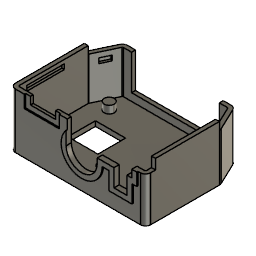
logger_case_bottom (Autodesk Fusion 360 design; units mm, degrees)
part number: 2026-07-28-14-06-36-773
Autodesk Fusion 360 part; units mm, degrees
sketch "Skizze1" plane through (0, 0, 0) normal (0, 0, 1) x (1, 0, 0)
  line L0 (0, 0) -> (-54, 0)
  line L1 (-54, 0) -> (-54, 30)
  line L2 (-54, 30) -> (-49, 40.5)
  line L3 (-49, 40.5) -> (-5, 40.5)
  line L4 (-5, 40.5) -> (0, 30)
  line L5 (0, 30) -> (0, 0)
  dimension "d1" = 54
  dimension "d2" = 30
  dimension "d3" = 40.5
  dimension "d4" = 30
  dimension "d5" = 10.5
  dimension "d6" = 44
  dimension "d7" = 5
  dimension "d8" = 5
  constraint coincident L0.start L5.end
  constraint horizontal L0
  constraint perpendicular L0 L1
  constraint perpendicular L1 L3
  constraint perpendicular L0 L5
  measures "d1" distance of L0.start L0.end
  measures "d2" distance of L0.end L1.end
  measures "d3" distance of L0 L3
  measures "d4" distance of L0.start L4.end
  measures "d5" distance of L3 L4.end
  measures "d6" distance of L2.end L3.end
  measures "d7" distance of L1 L2.end
  measures "d8" distance of L3.end L5
extrude "Extrusion1" add sketch "Skizze1" along normal blind 2 makes body 1
fillet "Abrundung1" radius 2 1 edges at (-54, 0, 1) on bodies 1
fillet "Abrundung2" radius 2 1 edges at (0, 0, 1) on bodies 1
fillet "Abrundung3" radius 2 1 edges at (0, 30, 1) on bodies 1
fillet "Abrundung4" radius 2 1 edges at (-5, 40.5, 1) on bodies 1
fillet "Abrundung5" radius 2 1 edges at (-49, 40.5, 1) on bodies 1
fillet "Abrundung6" radius 2 1 edges at (-54, 30, 1) on bodies 1
sketch "Skizze2" plane through (0, 0, 2) normal (0, 0, 1) x (-1, 0, 0)
  arc A0 (53.8057, -30.408) -> (54, -29.5481) centre (52, -29.5481) ccw
  line L0 (54, -29.5481) -> (54, -2)
  arc A1 (54, -2) -> (52, 0) centre (52, -2) ccw
  line L1 (52, 0) -> (2, 0)
  arc A2 (2, 0) -> (0, -2) centre (2, -2) ccw
  line L2 (0, -2) -> (0, -29.5481)
  arc A3 (0, -29.5481) -> (0.1943, -30.408) centre (2, -29.5481) ccw
  line L3 (0.1943, -30.408) -> (4.4571, -39.3599)
  arc A4 (4.4571, -39.3599) -> (6.2628, -40.5) centre (6.2628, -38.5) ccw
  line L4 (6.2628, -40.5) -> (47.7372, -40.5)
  arc A5 (47.7372, -40.5) -> (49.5429, -39.3599) centre (47.7372, -38.5) ccw
  line L5 (49.5429, -39.3599) -> (53.8057, -30.408)
  line L6 (1.6389, -29.7201) -> (5.9017, -38.672)
  arc A6 (5.9017, -38.672) -> (6.2628, -38.9) centre (6.2628, -38.5) ccw
  line L7 (6.2628, -38.9) -> (47.7372, -38.9)
  arc A7 (47.7372, -38.9) -> (48.0983, -38.672) centre (47.7372, -38.5) ccw
  line L8 (48.0983, -38.672) -> (52.3611, -29.7201)
  arc A8 (52.3611, -29.7201) -> (52.4, -29.5481) centre (52, -29.5481) ccw
  line L9 (52.4, -29.5481) -> (52.4, -2)
  arc A9 (52.4, -2) -> (52, -1.6) centre (52, -2) ccw
  line L10 (52, -1.6) -> (2, -1.6)
  arc A10 (2, -1.6) -> (1.6, -2) centre (2, -2) ccw
  line L11 (1.6, -2) -> (1.6, -29.5481)
  arc A11 (1.6, -29.5481) -> (1.6389, -29.7201) centre (2, -29.5481) ccw
  dimension "d23" = -1.6
extrude "Extrusion2" add sketch "Skizze2" along normal blind 20 bodies 1
sketch "Skizze3" plane through (0, 0, 0) normal (0, -1, 0) x (1, 0, 0)
  line L0 (-52, 22) -> (-52, 0)
  line L1 (-52, 0) -> (-2, 0)
  line L2 (-52, 22) -> (-46.4, 22)
  line L3 (-46.4, 22) -> (-46.4, 19)
  line L4 (-46.4, 19) -> (-36.4, 19)
  line L5 (-36.4, 19) -> (-36.4, 22)
  line L6 (-36.4, 22) -> (-31.2, 22)
  line L7 (-31.2, 13) -> (-31.2, 22)
  circle A0 centre (-25, 13) radius 6.2
  line L8 (0, 18) -> (-5, 18)
  line L9 (-5, 18) -> (-5, 15)
  line L10 (-5, 15) -> (-6.9, 15)
  line L11 (-6.9, 15) -> (-6.9, 8)
  line L12 (-6.9, 8) -> (-12.1, 8)
  line L13 (-12.1, 8) -> (-12.1, 15)
  line L14 (-46.4, 22) -> (-36.4, 22)
  line L15 (-31.2, 22) -> (0, 22)
  line L16 (-18.8, 13) -> (-18.8, 15)
  line L17 (-18.8, 15) -> (-12.1, 15)
  line L18 (0, 22) -> (0, 18)
  line L19 (0, 0) -> (-54, 0)
  line L20 (-54, 22) -> (-54, 0)
  point P0 (-54, 22)
  dimension "d27" = 3
  dimension "d28" = 10
  dimension "d29" = 5.2
  dimension "d30" = 12.4
  dimension "d31" = 13
  dimension "d32" = 9
  dimension "d33" = 6.2
  dimension "d36" = 19
  dimension "d37" = 4
  dimension "d40" = 5
  dimension "d41" = 3
  dimension "d42" = 1.9
  dimension "d43" = 7
  dimension "d44" = 5.2
  dimension "d45" = 7
  dimension "d123" = 7.6
  dimension "d127" = 6.2
  dimension "d129" = 6.7
  dimension "d131" = 10
  dimension "d132" = 31.2
  dimension "d150" = 22
  dimension "d151" = 18.8
  dimension "d152" = 22.8
  dimension "d154" = 8
  constraint coincident L0.start L2.start
  constraint perpendicular L2 L3
  constraint perpendicular L3 L4
  constraint perpendicular L6 L7
  constraint perpendicular L8 L9
  constraint perpendicular L9 L10
  constraint perpendicular L10 L11
  constraint perpendicular L11 L12
  constraint perpendicular L12 L13
  constraint parallel L6 L14
  constraint coincident A0 L16.start
  constraint vertical L16
  constraint parallel L15 L19
  constraint parallel L6 L19
  constraint parallel L2 L19
  constraint parallel L15 L17
  constraint parallel L12 L19
  constraint parallel L9 L18
  measures "d27" distance of L2.end L3.end
  measures "d28" distance of L3.end L4.end
  measures "d29" distance of L5.end L6.end
  measures "d30" diameter of A0
  measures "d31" distance of L1 A0.centre
  measures "d32" distance of L6.end L7.start
  measures "d33" distance of L7.start A0.centre
  measures "d36" distance of L1 L4
  measures "d37" distance of L8.start L15.end
  measures "d40" distance of L8.start L8.end
  measures "d41" distance of L8.end L9.end
  measures "d42" distance of L9.end L10.end
  measures "d43" distance of L10.end L11.end
  measures "d44" distance of L11.end L12.end
  measures "d45" distance of L12.end L13.end
  measures "d123" distance of L3 P0
  measures "d127" distance of A0.centre L16
  measures "d129" horizontal distance of L13.end L16.end
  measures "d131" horizontal distance of L2.end L5.end
  measures "d132" distance of L6.end L15.end
  measures "d150" distance of L0.start L0.end
  measures "d151" distance of L16.start L18
  measures "d152" distance of L7.start L20
  measures "d154" distance of L12 L19
extrude "Extrusion3" cut sketch "Skizze3" against normal blind 4 contours L7 A0 L8 L9 L10 L11 L12 L13 L15 L16 L17 L18 bodies 1
extrude "Extrusion4" cut sketch "Skizze3" against normal blind 3 contours A0 bodies 1
extrude "Extrusion5" cut sketch "Skizze3" against normal blind 3 contours L3 L4 L5 L14 bodies 1
sketch "Skizze4" plane through (0, 40.5, 0) normal (0, 1, 0) x (-1, 0, 0)
  line L0 (47.7372, 0) -> (47.7372, 22)
  line L1 (47.7372, 22) -> (6.2628, 22)
  line L2 (6.2628, 22) -> (6.2628, 0)
  line L3 (6.2628, 0) -> (47.7372, 0)
  line L4 (9.4998, 5) -> (44.4998, 5)
  line L5 (44.4998, 5) -> (44.4998, 22)
  line L6 (9.4998, 22) -> (44.4998, 22)
  line L7 (9.4998, 5) -> (9.4998, 22)
  line L8 (49, 0) -> (5, 0)
  line L9 (54.0455, 0) -> (54.0455, 22) construction
  line L10 (0.0455, 22) -> (0.0455, 0) construction
  point P0 (4.4571, 22)
  dimension "d56" = 17
  dimension "d57" = 35
  dimension "d58" = 3.237
  dimension "d59" = 3.2374
  dimension "d122" = 5
  dimension "d148" = 9.4543
  dimension "d149" = 9.5457
  constraint coincident L1 L6.start
  constraint perpendicular L2 L4
  constraint coincident L1 L5.end
  constraint perpendicular L1 L5
  constraint perpendicular L6 L7
  measures "d56" distance of L4.end L5.end
  measures "d57" distance of L4.start L4.end
  measures "d58" distance of L1.end L6.start
  measures "d59" distance of L0.end L5.end
  measures "d122" distance of L4 L8
  measures "d148" distance of L7 L10
  measures "d149" distance of L5 L9
extrude "Extrusion6" cut sketch "Skizze4" against normal blind 3 contours L1 L4 L5 L6 L7 bodies 1
sketch "Skizze5" plane through (0, 0, 22) normal (0, 0, 1) x (-1, 0, 0)
  line L0 (9.4998, -40.5) -> (9.4998, -38.9)
  line L1 (9.4998, -38.9) -> (6.2628, -38.9)
  arc A0 (5.9017, -38.672) -> (6.2628, -38.9) centre (6.2628, -38.5) ccw
  arc A1 (1.6, -29.5481) -> (1.6389, -29.7201) centre (2, -29.5481) ccw
  line L2 (1.6, -29.5481) -> (1.6, -4)
  line L3 (0, -4) -> (0, -29.5481)
  arc A2 (0, -29.5481) -> (0.1943, -30.408) centre (2, -29.5481) ccw
  line L4 (0.1943, -30.408) -> (4.4571, -39.3599)
  arc A3 (4.4571, -39.3599) -> (6.2628, -40.5) centre (6.2628, -38.5) ccw
  line L5 (6.2628, -40.5) -> (9.4998, -40.5)
  arc A4 (0, -29.5481) -> (0.1943, -30.408) centre (2, -29.5481) ccw
  line L6 (0.1943, -30.408) -> (4.4571, -39.3599)
  line L7 (49.5429, -39.3599) -> (53.8057, -30.408)
  arc A5 (53.8057, -30.408) -> (54, -29.5481) centre (52, -29.5481) ccw
  line L8 (44.4998, -40.5) -> (9.4998, -40.5)
  line L9 (44.4998, -40.5) -> (47.7372, -40.5)
  arc A6 (47.7372, -40.5) -> (49.5429, -39.3599) centre (47.7372, -38.5) ccw
  line L10 (6.2628, -40.5) -> (9.4998, -40.5)
  arc A7 (4.4571, -39.3599) -> (6.2628, -40.5) centre (6.2628, -38.5) ccw
  line L11 (54, -29.5481) -> (0, -29.5481)
  arc A8 (0, -29.5481) -> (0.1943, -30.408) centre (2, -29.5481) ccw
  line L12 (4.4571, -39.3599) -> (0.1943, -30.408)
  line L13 (1.6, -4) -> (0, -4)
  point P0 (0, -29.5481)
  constraint coincident A5.end L11.start
  constraint coincident P0 L3.end
extrude "Extrusion7" cut sketch "Skizze5" against normal blind 3 contours A2 L4 A3 L5 A4 L6 L7 A5 L8 L9 A6 L10 A7 L11 A8 L12 bodies 1
sketch "Skizze6" plane through (0, 0, 2) normal (0, 0, 1) x (-1, 0, 0)
  line L0 (1.6389, -29.7201) -> (5.9017, -38.672)
  arc A0 (5.9017, -38.672) -> (6.2628, -38.9) centre (6.2628, -38.5) ccw
  line L1 (6.2628, -38.9) -> (47.7372, -38.9)
  arc A1 (47.7372, -38.9) -> (48.0983, -38.672) centre (47.7372, -38.5) ccw
  line L2 (48.0983, -38.672) -> (52.3611, -29.7201)
  arc A2 (52.3611, -29.7201) -> (52.4, -29.5481) centre (52, -29.5481) ccw
  line L3 (52.4, -29.5481) -> (52.4, -2)
  arc A3 (52.4, -2) -> (52, -1.6) centre (52, -2) ccw
  line L4 (52, -1.6) -> (2, -1.6)
  arc A4 (2, -1.6) -> (1.6, -2) centre (2, -2) ccw
  line L5 (1.6, -2) -> (1.6, -29.5481)
  arc A5 (1.6, -29.5481) -> (1.6389, -29.7201) centre (2, -29.5481) ccw
  line L6 (45, -25) -> (33, -25)
  line L7 (33, -25) -> (33, -14)
  line L8 (33, -14) -> (45, -14)
  line L9 (45, -14) -> (45, -25)
  line L10 (44.4998, -40.5) -> (9.4998, -40.5)
  line L11 (36.4, 0) -> (46.4, 0)
  dimension "d65" = 12
  dimension "d66" = 11
  dimension "d69" = 15.5
  dimension "d70" = 14
  constraint horizontal L6
  constraint vertical L7
  constraint horizontal L8
  constraint vertical L9
  measures "d65" distance of L6.start L6.end
  measures "d66" distance of L6.start L8.end
  measures "d69" distance of L6 L10
  measures "d70" distance of L8 L11
extrude "Extrusion8" cut sketch "Skizze6" against normal blind 3 contours L6 L7 L8 L9 bodies 1
sketch "Skizze7" plane through (0, 0, 2) normal (0, 0, 1) x (-1, 0, 0)
  line L0 (33, -25) -> (33, -14)
  line L1 (33, -14) -> (45, -14)
  line L2 (45, -14) -> (45, -25)
  line L3 (45, -25) -> (33, -25)
  line L4 (1.6389, -29.7201) -> (5.9017, -38.672)
  arc A0 (5.9017, -38.672) -> (6.2628, -38.9) centre (6.2628, -38.5) ccw
  line L5 (6.2628, -38.9) -> (47.7372, -38.9)
  arc A1 (47.7372, -38.9) -> (48.0983, -38.672) centre (47.7372, -38.5) ccw
  line L6 (48.0983, -38.672) -> (52.3611, -29.7201)
  arc A2 (52.3611, -29.7201) -> (52.4, -29.5481) centre (52, -29.5481) ccw
  line L7 (52.4, -29.5481) -> (52.4, -2)
  arc A3 (52.4, -2) -> (52, -1.6) centre (52, -2) ccw
  line L8 (52, -1.6) -> (2, -1.6)
  arc A4 (2, -1.6) -> (1.6, -2) centre (2, -2) ccw
  line L9 (1.6, -2) -> (1.6, -29.5481)
  arc A5 (1.6, -29.5481) -> (1.6389, -29.7201) centre (2, -29.5481) ccw
  circle A6 centre (46, -31.5) radius 2
  line L10 (54, -29.5481) -> (54, -2)
  line L11 (44.4998, -40.5) -> (9.4998, -40.5)
  circle A7 centre (8, -31.5) radius 2
  line L12 (0, -4) -> (0, -29.5481)
  circle A8 centre (25, -8) radius 2
  line L13 (18.8, 0) -> (31.2, 0)
  dimension "d73" = 4
  dimension "d74" = 8
  dimension "d75" = 9
  dimension "d76" = 4
  dimension "d77" = 9
  dimension "d78" = 8
  dimension "d79" = 4
  dimension "d80" = 25
  dimension "d81" = 29
  dimension "d82" = 8
  measures "d73" diameter of A6
  measures "d74" distance of A6.centre L10
  measures "d75" distance of A6.centre L11
  measures "d76" diameter of A7
  measures "d77" distance of L11 A7.centre
  measures "d78" distance of A7.centre L12
  measures "d79" diameter of A8
  measures "d80" distance of L12 A8.centre
  measures "d81" distance of L10 A8.centre
  measures "d82" distance of A8.centre L13
extrude "Extrusion17" add sketch "Skizze7" along normal blind 3 separate body contours A6 | A7 | A8 makes body 2 at (-26.9975, 8.0997, 4) makes body 3 at (-9.9975, 31.5997, 4) makes body 4 at (-47.9975, 31.5997, 4)
sketch "Skizze8" plane through (0, 0, 0) normal (0, -1, 0) x (1, 0, 0)
  line L0 (-46.4, 19) -> (-46.4, 22)
  line L1 (-46.4, 22) -> (-52, 22)
  line L2 (-52, 22) -> (-52, 0)
  line L3 (-5, 18) -> (-5, 15)
  line L4 (-5, 15) -> (-6.9, 15)
  line L5 (-6.9, 15) -> (-6.9, 8)
  line L6 (-6.9, 8) -> (-12.1, 8)
  line L7 (-12.1, 8) -> (-12.1, 15)
  arc A0 (-31.2, 13) -> (-18.8, 13) centre (-25, 13) ccw
  line L8 (-36.4, 22) -> (-36.4, 19)
  line L9 (-36.4, 19) -> (-46.4, 19)
  arc A1 (-31.2, 13) -> (-18.8, 13) centre (-25, 13) ccw
  line L10 (-12.1, 8) -> (-12.1, 15)
  line L11 (-6.9, 8) -> (-12.1, 8)
  line L12 (-6.9, 15) -> (-6.9, 8)
  line L13 (-5, 15) -> (-6.9, 15)
  line L14 (-5, 18) -> (-5, 15)
  line L15 (-5, 18) -> (-3, 18)
  line L16 (-12.1, 15) -> (-18.8, 15)
  line L17 (-18.8, 15) -> (-18.8, 13)
  line L18 (-3, 18) -> (-3, 13)
  line L19 (-3, 13) -> (-4.9, 13)
  line L20 (-4.9, 13) -> (-4.9, 6)
  line L21 (-4.9, 6) -> (-14.1, 6)
  line L22 (-14.1, 6) -> (-14.1, 13)
  line L23 (-14.1, 13) -> (-16.8, 13)
  arc A2 (-33.2, 13) -> (-16.8, 13) centre (-25, 13) ccw
  circle A3 centre (-25, 13) radius 8.2
  line L24 (-31.2, 13) -> (-31.2, 18.3666)
  dimension "d85" = -2
  dimension "d155" = 16.4
  constraint coincident L3.start L14.start
  constraint perpendicular L15 L18
  constraint coincident A0.centre A1.centre
  constraint coincident A0.start A1.start
  constraint coincident A3 L24.end
  constraint tangent A1 L24
  constraint vertical L24
  measures "d155" diameter of A3
extrude "Extrusion10" add sketch "Skizze8" along normal blind 0.5 contours L3 L4 L5 L6 L7 L10 L11 L12 L13 L14 L15 L16 L18 L19 L20 L21 L22 L23 A3 bodies 1
extrude "Extrusion18" add sketch "Skizze8" along normal blind 0.5 contours A0 A1 L16 L17 A2 A3 L24 bodies 1
sketch "Skizze9" plane through (0, 0, 0) normal (0, -1, 0) x (1, 0, 0)
  line L0 (-36.4, 19) -> (-46.4, 19)
  line L1 (-46.4, 19) -> (-46.4, 22)
  line L2 (-36.4, 22) -> (-36.4, 19)
  line L3 (-34.4, 22) -> (-34.4, 17)
  line L4 (-34.4, 17) -> (-48.4, 17)
  line L5 (-48.4, 17) -> (-48.4, 22)
  line L6 (-48.4, 22) -> (-46.4, 22)
  line L7 (-36.4, 22) -> (-34.4, 22)
  dimension "d145" = -2
  constraint perpendicular L1 L6
  constraint perpendicular L3 L7
extrude "Extrusion11" cut sketch "Skizze9" against normal blind 0.5 bodies 1
sketch "Skizze10" plane through (-52.4, 0, 0) normal (1, 0, 0) x (0, 1, 0)
  line L0 (2, 2) -> (29.5481, 2)
  line L1 (29.5481, 2) -> (29.5481, 19)
  line L2 (29.5481, 19) -> (29.5481, 22)
  line L3 (29.5481, 22) -> (2, 22)
  line L4 (2, 22) -> (2, 2)
  line L5 (5, 20.5) -> (20, 20.5)
  line L6 (20, 20.5) -> (20, 18.5)
  line L7 (20, 18.5) -> (5, 18.5)
  line L8 (5, 18.5) -> (5, 20.5)
  dimension "d93" = 15
  dimension "d94" = 2
  dimension "d95" = 1.5
  dimension "d96" = 3
  constraint horizontal L5
  constraint vertical L6
  constraint horizontal L7
  constraint vertical L8
  measures "d93" distance of L6.end L7.end
  measures "d94" distance of L5.start L7.end
  measures "d95" distance of L3 L5
  measures "d96" distance of L4 L8
extrude "Extrusion13" cut sketch "Skizze10" against normal blind 1 contours L5 L6 L7 L8 bodies 1
sketch "Skizze11" plane through (-1.6, 0, 0) normal (-1, 0, 0) x (0, -1, 0)
  line L0 (-2, 18) -> (-4, 18)
  line L1 (-4, 18) -> (-4, 22)
  line L2 (-4, 22) -> (-29.5481, 22)
  line L3 (-29.5481, 22) -> (-29.5481, 19)
  line L4 (-29.5481, 19) -> (-29.5481, 2)
  line L5 (-29.5481, 2) -> (-2, 2)
  line L6 (-2, 2) -> (-2, 18)
  line L7 (-22, 20.5) -> (-7, 20.5)
  line L8 (-7, 20.5) -> (-7, 18.5)
  line L9 (-7, 18.5) -> (-22, 18.5)
  line L10 (-22, 18.5) -> (-22, 20.5)
  dimension "d100" = 15
  dimension "d102" = 2
  dimension "d103" = 3
  dimension "d104" = 1.5
  constraint horizontal L7
  constraint vertical L8
  constraint horizontal L9
  constraint vertical L10
  measures "d100" distance of L8.end L9.end
  measures "d102" distance of L7.start L9.end
  measures "d103" distance of L1 L8
  measures "d104" distance of L2 L7
extrude "Extrusion14" cut sketch "Skizze11" against normal blind 1 contours L7 L8 L9 L10 bodies 1
sketch "Skizze12" plane through (-54.219, 25.8186, 0) normal (0.902861, -0.429934, 0) x (0.429934, 0.902861, 0)
  line L0 (14.2363, 19) -> (4.3213, 19)
  line L1 (4.3213, 19) -> (4.3213, 2)
  line L2 (4.3213, 2) -> (14.2363, 2)
  line L3 (14.2363, 2) -> (14.2363, 19)
  line L4 (7.3213, 17) -> (11.3213, 17)
  line L5 (11.3213, 17) -> (11.3213, 15)
  line L6 (11.3213, 15) -> (7.3213, 15)
  line L7 (7.3213, 15) -> (7.3213, 17)
  dimension "d107" = 4
  dimension "d108" = 2
  dimension "d109" = 3
  dimension "d110" = 2.915
  dimension "d111" = 2
  constraint horizontal L4
  constraint vertical L5
  constraint horizontal L6
  constraint vertical L7
  measures "d107" distance of L5.end L6.end
  measures "d108" distance of L4.start L6.end
  measures "d109" distance of L1 L7
  measures "d110" distance of L3 L5
  measures "d111" distance of L0 L4
extrude "Extrusion15" cut sketch "Skizze12" against normal blind 1 contours L4 L5 L6 L7 bodies 1
sketch "Skizze13" plane through (10.2005, 4.8574, 0) normal (-0.902861, -0.429934, 0) x (0.429934, -0.902861, 0)
  line L0 (-27.5377, 19) -> (-37.4527, 19)
  line L1 (-37.4527, 19) -> (-37.4527, 2)
  line L2 (-37.4527, 2) -> (-27.5377, 2)
  line L3 (-27.5377, 2) -> (-27.5377, 19)
  line L4 (-34.5377, 17) -> (-30.5377, 17)
  line L5 (-30.5377, 17) -> (-30.5377, 15)
  line L6 (-30.5377, 15) -> (-34.5377, 15)
  line L7 (-34.5377, 15) -> (-34.5377, 17)
  dimension "d114" = 4
  dimension "d115" = 2
  dimension "d116" = 2
  dimension "d117" = 3
  constraint horizontal L4
  constraint vertical L5
  constraint horizontal L6
  constraint vertical L7
  measures "d114" distance of L5.end L6.end
  measures "d115" distance of L4.start L6.end
  measures "d116" distance of L0 L4
  measures "d117" distance of L3 L5
extrude "Extrusion16" cut sketch "Skizze13" against normal blind 1 contours L4 L5 L6 L7 bodies 1
